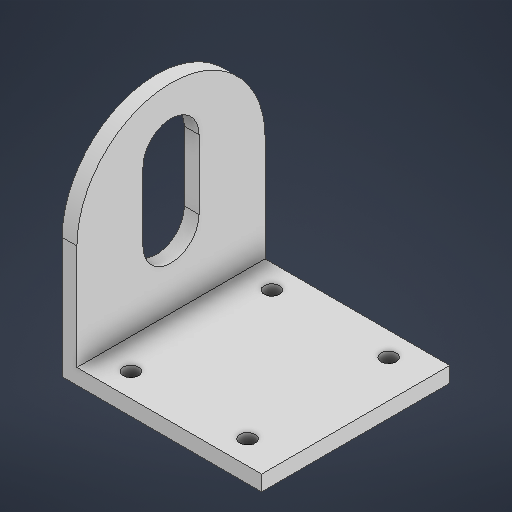
# Autodesk Inventor part: Drive Motor Stand
Saved by Autodesk Inventor 2026.3 (Build 303398000, 398)
## iProperties
Created: 2026-06-06
Part Number: Drive Motor Stand
Material: Generic
Document SubType Name: Modeling
Designer: Inigo Greenall
Density: 1 g/cm^3
Appearance: Default
Mass: 9.52169 g
Surface Area: 69.9605 cm^2
Volume: 9.52169 cm^3
Author: Inigo Greenall
Autodesk Inventor part; units mm, degrees
ref_plane "YZ Plane" through (0, 0, 0) normal (1, 0, 0) x (0, 1, 0)
ref_plane "XZ Plane" through (0, 0, 0) normal (0, 1, 0) x (-1, 0, 0)
ref_plane "XY Plane" through (0, 0, 0) normal (0, 0, 1) x (1, 0, 0)
sketch "Sketch1" plane through (0, 0, 0) normal (0, 1, 0) x (-1, 0, 0)
  line L0 (21.35, -20.15) -> (-21.35, -20.15)
  line L1 (-21.35, -20.15) -> (-21.35, 20.15)
  line L2 (-21.35, 20.15) -> (21.35, 20.15)
  line L3 (21.35, 20.15) -> (21.35, -20.15)
  circle A0 centre (-13.3, -15.1) radius 1.65
  circle A1 centre (11.7, -15.1) radius 1.65
  circle A2 centre (-13.3, 15.1) radius 1.65
  circle A3 centre (11.7, 15.1) radius 1.65
  point P0 (0, 0)
  point P1 (0, -20.15)
  point P2 (21.35, 0)
  dimension "d0" = 40.3
  dimension "d1" = 42.7
  dimension "d2" = 6.4
  dimension "d3" = 3.3
  dimension "d4" = 3.4
  dimension "d7" = 25
  dimension "d10" = 30.2
  constraints: 8 end point, 4 centre point, 2 horizontal, 2 midpoint, 2 parallel, 1 horizontal alignment, 1 perpendicular, 1 vertical, 1 vertical alignment, 6 other
  measures "d0" distance of L2.end L0.start
  measures "d1" distance of L0.start L0.end
  measures "d2" distance edge to line of A0 L1
  measures "d3" diameter of A0
  measures "d4" distance edge to line of A0 L0
  measures "d7" distance of A0.centre A1.centre
  measures "d10" distance of A0.centre A2.centre
extrude "Extrusion1" add sketch "Sketch1" along normal blind 3.3
sketch "Sketch2" plane through (0, 3.3, 0) normal (0, 1, 0) x (1, 0, 0)
  line L0 (-21.35, 20.15) -> (-21.35, -20.15) projected
  line L1 (-21.35, -20.15) -> (21.35, -20.15) projected
  line L2 (-21.35, 20.15) -> (-18.2, 20.15)
  line L3 (-18.2, 20.15) -> (-18.2, -20.15)
  line L4 (-18.2, -20.15) -> (-21.35, -20.15)
  line L5 (-21.35, -20.15) -> (-21.35, 20.15)
  point P0 (0, 0)
  dimension "d15" = 3.15
  constraints: 8 end point, 2 parallel, 1 horizontal, 1 perpendicular, 1 point on line
  measures "d15" distance between parallel lines of L3 L0
extrude "Extrusion2" add sketch "Sketch2" along normal blind 42.7
sketch "Sketch3" plane through (-21.35, 0, -20.15) normal (-1, 0, 0) x (0, 0, 1)
  line L0 (40.3, 3.3) -> (40.3, 46) projected
  line L1 (0, 3.3) -> (0, 46) projected
  arc A0 (40.3, 25.85) -> (0, 25.85) centre (20.15, 25.85) ccw
  line L2 (0, 46) -> (40.3, 46) projected
  point P0 (20.15, 0)
  point P1 (20.15, 46)
  point P2 (0, 31.0213)
  point P3 (40.3, 31.0213)
  constraints: 3 point on circle, 2 point on line, 1 centre point, 1 midpoint, 1 tangent
extrude "Extrusion3" cut sketch "Sketch3" against normal through all
sketch "Sketch4" plane through (-21.35, 0, -20.15) normal (-1, 0, 0) x (0, 0, 1)
  arc A0 (26.15, 33.4) -> (14.15, 33.4) centre (20.15, 33.4) ccw
  line L0 (14.15, 33.4) -> (14.15, 18.6)
  line L1 (26.15, 33.4) -> (26.15, 18.6)
  arc A1 (14.15, 18.6) -> (26.15, 18.6) centre (20.15, 18.6) ccw
  arc A2 (40.3, 25.85) -> (0, 25.85) centre (20.15, 25.85) ccw projected
  point P0 (20.15, 0)
  point P1 (20.15, 46)
  point P2 (20.15, 39.4)
  point P3 (20.15, 46)
  point P4 (20.15, 12.6)
  dimension "d20" = 6.6
  dimension "d21" = 6
  dimension "d22" = 26.8
  constraints: 8 point on circle, 4 end point, 4 tangent, 2 centre point, 2 vertical, 1 vertical alignment
  measures "d20" distance of point (20.15, 46) point (20.15, 39.4)
  measures "d21" radius of A0
  measures "d22" distance of point (20.15, 12.6) point (20.15, 39.4)
extrude "Extrusion4" cut sketch "Sketch4" against normal through all
body "Solid1"
